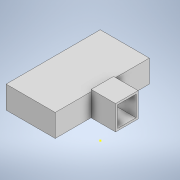
# Autodesk Inventor part: tof-mount
Saved by Autodesk Inventor 2022 (Build 260153000, 153)
## iProperties
Created: 2023-04-06
Part Number: tof-mount
Material: Generic
Document SubType Name: Modeling
Designer: Hamza Siddiqui
Density: 1 g/cm^3
Appearance: Default
Author: Hamza Siddiqui
Autodesk Inventor part; units mm, degrees
ref_plane "YZ Plane" through (0, 0, 0) normal (1, 0, 0) x (0, 1, 0)
ref_plane "XZ Plane" through (0, 0, 0) normal (0, 1, 0) x (-1, 0, 0)
ref_plane "XY Plane" through (0, 0, 0) normal (0, 0, 1) x (1, 0, 0)
sketch "Sketch1" plane through (0, 0, 0) normal (0, 1, 0) x (-1, 0, 0)
  line L0 (0, -3.6919) -> (0, -9.1919)
  line L1 (0, -9.1919) -> (6, -9.1919)
  line L2 (0, -3.6919) -> (6, -3.6919)
  line L3 (6, -3.6919) -> (6, 3.0581)
  line L4 (6, 3.0581) -> (18, 3.0581)
  line L5 (18, 3.0581) -> (18, -15.9419)
  line L6 (18, -15.9419) -> (6, -15.9419)
  line L7 (6, -15.9419) -> (6, -9.1919)
  point P0 (0, 0)
  dimension "d0" = 5.5
  dimension "d1" = 6
  dimension "d3" = 12
  dimension "d4" = 6.75
  dimension "d5" = 6.75
  dimension "d6" = 19
  dimension "d7" = 12
  constraints: 16 end point, 3 perpendicular, 2 vertical, 1 horizontal, 1 point on line
  measures "d0" distance of L0.start L0.end
  measures "d1" distance of L0.end L1.end
  measures "d3" distance of L5.end L6.end
  measures "d4" distance of L6.end L1.end
  measures "d5" distance of L2.end L3.end
  measures "d6" distance of L4.end L5.end
  measures "d7" distance of L3.end L4.end
sketch "Sketch2" plane through (0, 0, 0) normal (0, 1, 0) x (-1, 0, 0)
  point P0 (0, 0)
extrude "Extrusion1" add sketch "Sketch1" along normal blind 6
sketch "Sketch3" plane through (0, 6, 0) normal (0, 1, 0) x (1, 0, 0)
  line L0 (-6, 15.9419) -> (-18, 15.9419) projected
  line L1 (-6, -3.0581) -> (-6, 3.6919) projected
  line L2 (-18, 15.9419) -> (-6, 15.9419)
  line L3 (-6, 15.9419) -> (-6, -3.0581)
  line L4 (-6, -3.0581) -> (-18, -3.0581)
  line L5 (-18, -3.0581) -> (-18, 15.9419)
  point P0 (0, 0)
  constraints: 8 end point, 2 parallel, 1 horizontal, 1 perpendicular
extrude "Extrusion2" cut sketch "Sketch3" against normal blind 2
sketch "Sketch4" plane through (-18, 0, -15.9419) normal (-1, 0, 0) x (0, 0, 1)
  point P0 (15.9419, 0)
sketch "Sketch5" plane through (-18, 0, 3.0581) normal (0, 0, 1) x (1, 0, 0)
  line L0 (12, 4) -> (0, 4) projected
  line L1 (0, 0) -> (12, 0) projected
  line L2 (12, 4) -> (0, 4)
  line L3 (0, 4) -> (0, 0)
  line L4 (0, 0) -> (12, 0)
  line L5 (12, 0) -> (12, 4)
  point P0 (18, 0)
  constraints: 8 end point, 2 parallel, 1 horizontal, 1 perpendicular
extrude "Extrusion3" add sketch "Sketch5" along normal blind 2
sketch "Sketch6" plane through (-6, 0, -15.9419) normal (0, 0, -1) x (-1, 0, 0)
  line L0 (12, 4) -> (0, 4) projected
  line L1 (0, 0) -> (12, 0) projected
  line L2 (0, 4) -> (12, 4)
  line L3 (12, 4) -> (12, 0)
  line L4 (12, 0) -> (0, 0)
  line L5 (0, 0) -> (0, 4)
  point P0 (-6, 0)
  constraints: 8 end point, 2 parallel, 1 horizontal, 1 perpendicular
extrude "Extrusion4" add sketch "Sketch6" along normal blind 2
sketch "Sketch7" plane through (-18, 0, 5.0581) normal (-1, 0, 0) x (0, 0, 1)
  point P0 (-5.0581, 0)
sketch "Sketch8" plane through (-18, 0, 5.0581) normal (-1, 0, 0) x (0, 0, 1)
  point P0 (-5.0581, 0)
sketch "Sketch9" plane through (0, 4, 0) normal (0, 1, 0) x (1, 0, 0)
  line L0 (-18, -5.0581) -> (-6, -5.0581) projected
  line L1 (-6, 9.1919) -> (-6, 17.9419) projected
  line L2 (-18, -5.0581) -> (-6, -5.0581)
  line L3 (-6, -5.0581) -> (-6, 17.9419)
  line L4 (-6, 17.9419) -> (-18, 17.9419)
  line L5 (-18, 17.9419) -> (-18, -5.0581)
  point P0 (0, 0)
  constraints: 8 end point, 2 parallel, 1 horizontal, 1 perpendicular
extrude "Extrusion5" add sketch "Sketch9" along normal blind 1.5
sketch "Sketch10" plane through (-18, 0, -17.9419) normal (-1, 0, 0) x (0, 0, 1)
  line L0 (1.5, 1) -> (21.5, 1)
  line L1 (21.5, 1) -> (21.5, 4.5)
  line L2 (21.5, 4.5) -> (1.5, 4.5)
  line L3 (1.5, 4.5) -> (1.5, 1)
  line L4 (0, 5.5) -> (23, 5.5) projected
  line L5 (23, 0) -> (0, 0) projected
  line L6 (0, 0) -> (0, 5.5) projected
  line L7 (23, 0) -> (23, 5.5) projected
  point P0 (17.9419, 0)
  dimension "d22" = 1
  dimension "d23" = 1
  dimension "d24" = 1.5
  dimension "d25" = 1.5
  constraints: 8 end point, 2 parallel, 1 horizontal, 1 perpendicular
  measures "d22" distance between parallel lines of L2 L4
  measures "d23" distance between parallel lines of L5 L0
  measures "d24" distance between parallel lines of L6 L3
  measures "d25" distance between parallel lines of L7 L1
extrude "Extrusion6" cut sketch "Sketch10" against normal blind 10 contours L3 L2 L1 L0
sketch "Sketch11" plane through (0, 0, -3.6919) normal (1, 0, 0) x (0, 0, -1)
  line L0 (14.25, 5.5) -> (-8.75, 5.5) projected
  line L1 (5, 5.5) -> (0.5, 5.5)
  line L2 (0.5, 5.5) -> (0.5, 0.5)
  line L3 (0.5, 0.5) -> (5, 0.5)
  line L4 (5, 0.5) -> (5, 5.5)
  line L5 (0, 0) -> (5.5, 0) projected
  line L6 (0, 0) -> (0, 6) projected
  line L7 (5.5, 0) -> (5.5, 6) projected
  point P0 (-3.6919, 0)
  point P1 (0.5, 5.5)
  dimension "d28" = 0.5
  dimension "d29" = 0.5
  dimension "d30" = 0.5
  constraints: 8 end point, 2 parallel, 1 horizontal, 1 perpendicular, 1 point on line
  measures "d28" distance between parallel lines of L5 L3
  measures "d29" distance between parallel lines of L6 L2
  measures "d30" distance between parallel lines of L7 L4
extrude "Extrusion7" cut sketch "Sketch11" against normal blind 6 contours L4 L3 L2 L0
sketch "Sketch12" plane through (0, 0, 0) normal (0, -1, 0) x (1, 0, 0)
  point P0 (0, 0)
sketch "Sketch13" plane through (0, 0, 0) normal (0, -1, 0) x (1, 0, 0)
  point P0 (0, 0)
sketch "Sketch14" plane through (0, 0, 0) normal (0, -1, 0) x (1, 0, 0)
  point P0 (0, 0)
sketch "Sketch15" plane through (0, 0, 0) normal (0, -1, 0) x (1, 0, 0)
  line L0 (-17.25, -11.9419) -> (-6.75, -11.9419)
  line L1 (-6.75, -11.9419) -> (-6.75, -0.9419)
  line L2 (-6.75, -0.9419) -> (-17.25, -0.9419)
  line L3 (-17.25, -0.9419) -> (-17.25, -11.9419)
  line L4 (-6, -17.9419) -> (-18, -17.9419) projected
  line L5 (-18, 5.0581) -> (-6, 5.0581) projected
  line L6 (-18, 5.0581) -> (-18, -17.9419) projected
  line L7 (-6, -3.6919) -> (-6, 5.0581) projected
  point P0 (0, 0)
  dimension "d33" = 6
  dimension "d34" = 6
  dimension "d35" = 0.75
  dimension "d36" = 0.75
  constraints: 8 end point, 2 parallel, 1 horizontal, 1 perpendicular
  measures "d33" distance between parallel lines of L4 L0
  measures "d34" distance between parallel lines of L5 L2
  measures "d35" distance between parallel lines of L6 L3
  measures "d36" distance between parallel lines of L7 L1
extrude "Extrusion8" cut sketch "Sketch15" against normal up to surface (4.5 mm away)
body "Solid1"
